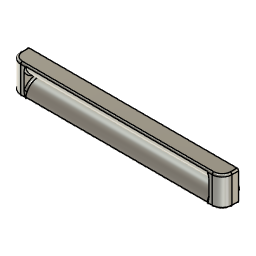
card_placeholder (Autodesk Fusion 360 design; units mm, degrees)
Autodesk Fusion 360 part; units mm, degrees
sketch "Sketch1" plane through (0, 0, 0) normal (0, 1, 0) x (1, 0, 0)
  line L0 (0, 0) -> (56, 0)
  line L1 (56, 0) -> (56, -1)
  line L2 (56, -1) -> (0, -1)
  line L3 (0, -1) -> (0, 0)
  line L4 (60, -5) -> (-4, -5)
  line L5 (-4, -5) -> (-4, 4)
  line L6 (-4, 4) -> (60, 4)
  line L7 (60, 4) -> (60, -5)
  dimension "d1" = 56
  dimension "d2" = 1
  dimension "d3" = -4
  constraint horizontal L0
  constraint vertical L1
  constraint horizontal L2
  constraint vertical L3
  constraint coincident L0.start L3.end
  measures "d1" distance of L0.start L0.end
  measures "d2" distance of L0.start L2.end
extrude "Extrude1" add sketch "Sketch1" along normal blind 8
fillet "Fillet1" radius 4 2 edges at (28, 0, 0) (28, 0, 1)
fillet "Fillet2" radius 3 2 edges at (60, 0, 0.5) (-4, 0, 0.5)
fillet "Fillet3" radius 0.5 7 edges at (28, 0, -4) (-4, 5.5, -4) (-3.1213, 0.8787, -4) (-0.5, 0, -4) (56.5, 0, -4) (59.1213, 0.8787, -4) (60, 5.5, -4)
fillet "Fillet4" radius 0.5 7 edges at (60, 5.5, 5) (59.1213, 0.8787, 5) (56.5, 0, 5) (28, 0, 5) (-0.5, 0, 5) (-3.1213, 0.8787, 5) (-4, 5.5, 5)
extrude "Extrude2" cut 1 faces at (18.6667, 8, 3.6667) along direction (0, -1, 0) blind 3
fillet "Fillet5" radius 0.5 2 edges at (56, 4.5, 1) (56, 1.3056, 2.0436)
fillet "Fillet6" radius 0.5 3 edges at (56, 0.1579, -3.8273) (56, 1.3814, -0.9763) (56, 4.5, 0)
fillet "Fillet7" radius 0.5 5 edges at (0, 1.3056, 2.0436) (0, 4.5, 1) (0, 4.5, 0) (0, 1.3814, -0.9763) (0, 0.1579, -3.8273)
sketch "Sketch2" plane through (0, 5, 0) normal (0, 1, 0) x (-1, 0, 0)
  arc A0 (-0.5, 0) -> (-0.5, 1) centre (-0.5, 0.5) ccw
  line L0 (-0.5, 0) -> (-55.5, 0)
  arc A1 (-55.5, 1) -> (-55.5, 0) centre (-55.5, 0.5) ccw
  line L1 (-55.5, 1) -> (-0.5, 1)
  arc A2 (4, 4.5) -> (3.5, 5) centre (3.5, 4.5) ccw
  line L2 (3.5, 5) -> (-59.5, 5)
  arc A3 (-59.5, 5) -> (-60, 4.5) centre (-59.5, 4.5) ccw
  line L3 (-60, 4.5) -> (-60, -3.5)
  arc A4 (-60, -3.5) -> (-59.5, -4) centre (-59.5, -3.5) ccw
  line L4 (-59.5, -4) -> (3.5, -4)
  arc A5 (3.5, -4) -> (4, -3.5) centre (3.5, -3.5) ccw
  line L5 (4, -3.5) -> (4, 4.5)
  circle A6 centre (-57, -2) radius 1.25
  line L6 (-28, -4) -> (-28, 8.2756) construction
  line L7 (-28, -4) -> (-28, 8.2756) construction
  circle A7 centre (1, -2) radius 1.25
  dimension "d22" = 2.5
  dimension "d24" = 3
  dimension "d25" = 2
  constraint midpoint L4 L6.start
  constraint perpendicular L1 L6
  constraint symmetric A6 L6 A7
  constraint symmetric L7.start L6 L6.start
  constraint symmetric L7.end L6 L6.end
  measures "d22" diameter of A6
  measures "d24" distance of L3 A6.centre
  measures "d25" distance of L4 A6.centre
extrude "Extrude3" add sketch "Sketch2" along normal blind 2 contours A6 | A7
